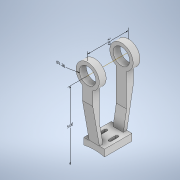
# Autodesk Inventor part: finderV02
Saved by Autodesk Inventor 2020.3 (Build 243373000, 373)
## iProperties
Created: 2020-06-03
Part Number: finderV02
Material: Generic
Document SubType Name: Modeling
Designer: robst
Density: 1 g/cm^3
Appearance: Default
Author: robst
Autodesk Inventor part; units mm, degrees
sketch "Sketch1" plane through (0, 0, 0) normal (0, 0, 1) x (1, 0, 0)
  arc A0 (19.05, 80.3219) -> (-19.05, 80.3219) centre (0, 0) ccw
  line L0 (0, 0) -> (0, 152.4) construction
  line L1 (0, 93.0219) -> (19.05, 93.0219)
  line L2 (19.05, 93.0219) -> (19.05, 80.3219)
  line L3 (0, 93.0219) -> (-19.05, 93.0219)
  line L4 (-19.05, 93.0219) -> (-19.05, 80.3219)
  dimension "telescopeTubeDiameter" = 165.1
  dimension "d1" = 152.4
  dimension "d2" = 19.05
  dimension "d3" = 12.7
  constraints: 10 end point, 2 point on circle, 2 symmetric about line, 1 centre point, 1 coincident, 1 horizontal, 1 perpendicular, 1 point on line, 1 vertical
  measures "telescopeTubeDiameter" diameter of A0
  measures "d1" distance of L0.start L0.end
  measures "d2" distance of L1.start L1.end
  measures "d3" distance of L1.end L2.end
extrude "Extrusion1" add sketch "Sketch1" along normal mid plane 50.8
sketch "Sketch2" plane through (-19.05, 93.0219, 25.4) normal (0, 1, 0) x (1, 0, 0)
  line L0 (38.1, 0) -> (0, 0) construction
  line L1 (19.05, 0) -> (19.05, 50.8) construction
  line L2 (0, 50.8) -> (38.1, 50.8) construction
  line L3 (0, 50.8) -> (0, 0) construction
  line L4 (0, 25.4) -> (38.1, 25.4) construction
  line L5 (38.1, 50.8) -> (38.1, 0) construction
  line L6 (29.21, 19.05) -> (29.21, 31.75) construction
  line L7 (31.75, 19.05) -> (31.75, 31.75)
  line L8 (26.67, 31.75) -> (26.67, 19.05)
  arc A0 (26.67, 19.05) -> (31.75, 19.05) centre (29.21, 19.05) ccw
  arc A1 (31.75, 31.75) -> (26.67, 31.75) centre (29.21, 31.75) ccw
  point P0 (19.05, 25.4)
  point P1 (29.21, 25.4)
  dimension "d6" = 0
  dimension "d7" = 10.16
  dimension "d8" = 6.35
  dimension "d11" = 5.08
  constraints: 12 end point, 5 midpoint, 4 point on circle, 4 tangent, 2 centre point, 2 parallel
  measures "d6" distance from line of point (29.21, 25.4) L4
  measures "d7" distance between parallel lines of L6 L1
  measures "d8" distance of L6.end point (29.21, 25.4)
  measures "d11" distance between parallel lines of L7 L8
extrude "Extrusion2" cut sketch "Sketch2" against normal through all
mirror "Mirror1" about plane through (0, 0, 0) normal (1, 0, 0) of "Extrusion2"
sketch "Sketch3" plane through (0, 0, 0) normal (1, 0, 0) x (0, 1, 0)
  line L0 (93.0219, 25.4) -> (93.0219, -25.4) projected
  line L1 (80.3219, -25.4) -> (93.0219, -25.4) projected
  line L2 (162.8719, -25.4) -> (162.8719, -37.137) construction
  line L3 (93.0219, -25.4) -> (162.8719, -37.7164)
  line L4 (93.0219, -25.4) -> (162.8719, -25.4) construction
  line L5 (93.0219, -18.952) -> (162.8719, -31.2685)
  line L6 (162.8719, -31.2685) -> (162.8719, -37.7164)
  point P0 (0, 0)
  dimension "d13" = 69.85
  dimension "d14" = 10
  dimension "d15" = 6.35
  constraints: 10 end point, 2 point on line, 1 midpoint, 1 parallel, 1 perpendicular, 1 vertical
  measures "d13" distance of L0.end L2.start
  measures "d14" angle of L3 L4
  measures "d15" distance between parallel lines of L5 L3
extrude "Extrusion3" add sketch "Sketch3" along normal mid plane 19.05
ref_plane "Work Plane1" through (9.525, 162.8719, -37.7164) normal (0, 0, 1) x (1, 0, 0)
sketch "Sketch4" plane through (9.525, 162.8719, -37.7164) normal (0, 0, 1) x (1, 0, 0)
  line L0 (0, 0) -> (-19.05, 0) projected
  line L1 (-19.05, 0) -> (0, 0) construction
  line L2 (-9.525, 0) -> (-9.525, 50.8) construction
  circle A0 centre (-9.525, 44.45) radius 15.24
  arc A1 (0, 25.0747) -> (-19.05, 25.0747) centre (-9.525, 44.45) ccw
  line L3 (0, 0) -> (0, 25.0747)
  line L4 (-19.05, 0) -> (-19.05, 25.0747)
  point P0 (-9.525, -162.8719)
  dimension "d18" = 50.8
  dimension "d19" = 30.48
  dimension "d20" = 6.35
  dimension "d25" = 44.45
  constraints: 6 end point, 2 centre point, 2 point on circle, 2 vertical, 1 coincident, 1 midpoint, 1 parallel, 1 point on line
  measures "d18" distance of L2.start L2.end
  measures "d19" diameter of A0
  measures "d20" radial gap between concentric circles of A1 A0
  measures "d25" distance from line of A0.centre L0
extrude "Extrusion4" add sketch "Sketch4" along normal blind 12.7
sketch "Sketch7" plane through (0, 0, 0) normal (1, 0, 0) x (0, 1, 0)
  line L0 (93.0219, -18.952) -> (162.8719, -31.2685) projected
  line L1 (162.8719, -31.2685) -> (162.8719, -25.0164) projected
  line L2 (162.8719, -25.0164) -> (127.4148, -25.0164)
  line L3 (127.4148, -25.0164) -> (162.8719, -31.2685)
  line L4 (187.9465, -25.0164) -> (162.8719, -25.0164) projected
  line L5 (162.8719, -31.2685) -> (162.8719, -25.0164)
  point P0 (0, 0)
  constraints: 6 end point, 1 collinear, 1 horizontal, 1 point on line, 1 vertical
extrude "Extrusion5" add sketch "Sketch7" along normal mid plane 19.05
mirror "Mirror4" about plane through (0, 0, 0) normal (0, 0, 1) of "Extrusion4", "Extrusion3"
sketch "Sketch8" plane through (0, 0, 0) normal (1, 0, 0) x (0, 1, 0)
  line L0 (162.8719, 31.2685) -> (162.8719, 25.0164) projected
  line L1 (93.0219, 18.952) -> (162.8719, 31.2685) projected
  line L2 (162.8719, 25.0164) -> (127.4148, 25.0164)
  line L3 (127.4148, 25.0164) -> (162.8719, 31.2685)
  line L4 (162.8719, 31.2685) -> (162.8719, 25.0164)
  point P0 (0, 0)
  constraints: 6 end point, 1 collinear, 1 horizontal, 1 point on line
extrude "Extrusion6" add sketch "Sketch8" along normal mid plane 19.05
ref_plane "Work Plane3" through (19.05, 80.3219, 25.4) normal (0, 1, 0) x (-1, 0, 0)
ref_plane "Work Plane4" through (0, 228.9119, -25.0164) normal (0, 1, 0) x (-1, 0, 0)
equation "\"d62\" = 0.125 * Sketch12_Pitch"
equation "\"Sketch12_Pitch\" = 0.79375"
equation "\"d64\" = 60deg"
equation "\"d101\" = 55deg"
equation "\"Sketch15_Pitch\" = 0.79375"
equation "\"d119\" = 55deg"
equation "\"Sketch17_Pitch\" = 0.79375"
equation "\"d137\" = 55deg"
equation "\"Sketch19_Pitch\" = 0.79375"
equation "\"d155\" = 55deg"
equation "\"Sketch21_Pitch\" = 0.79375"
equation "\"d173\" = 55deg"
equation "\"Sketch23_Pitch\" = 0.79375"
equation "\"d191\" = 55deg"
equation "\"Sketch25_Pitch\" = 0.79375"
body "Solid1"
